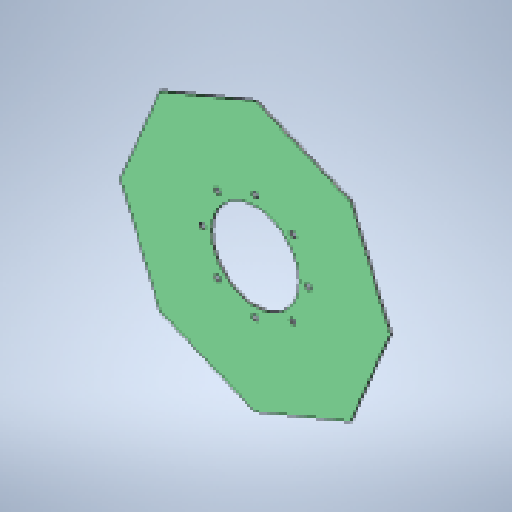
# Autodesk Inventor part: DMF 01 21 Барабан торец НОС v2.1_наруж
Saved by Autodesk Inventor 2026.2 (Build 302298010, 298A)
## iProperties
Created: 2024-04-28
Part Number: DMF 01 21 Барабан торец НОС v2.1_наруж
Material: Generic
Document SubType Name: Sheet Metal
Designer: admin
Stock Number: Барабан_Торец_Нос
Density: 1 g/cm^3
Flat Pattern Width: 51.5 cm
Flat Pattern Length: 51.5 cm
Flat Pattern Area: 2652.25 cm^2
Sheet Metal Rule: Default
Sheet Metal Width: 515,000 mm
Sheet Metal Length: 515,000 mm
Sheet Metal Area: 265225,000 mm^2
Appearance: Default
Author: pokla
Autodesk Inventor part; units mm, degrees
ref_plane "YZ Plane" through (0, 0, 0) normal (1, 0, 0) x (0, 1, 0)
ref_plane "XZ Plane" through (0, 0, 0) normal (0, 1, 0) x (-1, 0, 0)
ref_plane "XY Plane" through (0, 0, 0) normal (0, 0, 1) x (1, 0, 0)
sketch "Sketch2" plane through (0, 0, 0) normal (0, 0, 1) x (1, 0, 0)
  line L0 (-197.082, 197.082) -> (0, 278.716)
  line L1 (0, 278.716) -> (197.082, 197.082)
  line L2 (197.082, 197.082) -> (278.716, 0)
  line L3 (278.716, 0) -> (197.082, -197.082)
  line L4 (197.082, -197.082) -> (0, -278.716)
  line L5 (0, -278.716) -> (-197.082, -197.082)
  line L6 (-197.082, -197.082) -> (-278.716, 0)
  line L7 (-278.716, 0) -> (-197.082, 197.082)
  circle A0 centre (0, 0) radius 90
  dimension "d23" = 515
  dimension "d26" = 180
  measures "d23" distance between parallel lines of L6 L2
  measures "d26" diameter of A0
extrude "Plate1" add sketch "Sketch2" against normal blind 3
sketch "Sketch4" plane through (0, 0, 0) normal (0, 0, 1) x (1, 0, 0)
  circle A0 centre (0, 110) radius 6.25
  circle A1 centre (0, 0) radius 90 projected
  circle A2 centre (0, 0) radius 110 construction
  dimension "d28" = 220
  dimension "d16" = 12.5
  constraints: 2 vertical alignment, 1 centre point, 1 coincident, 2 other
  measures "d16" diameter of A0
extrude "Extrusion1" cut sketch "Sketch4" against normal up to surface (3 mm away) contours A0
pattern_circular "Circular Pattern1" count 8 over 360 about axis through (0, 0, -10) along (0, 0, 1) of "Extrusion1"
equation "\"d23\" = Барабан_размер_по_плоскостям"
equation "\"d15\" = Thickness"
equation "\"BendRadius\" = Thickness"
equation "\"BendReliefWidth\" = Thickness"
equation "\"BendReliefDepth\" = 0.5 * Thickness"
equation "\"CornerReliefSize\" = 4 * Thickness"
equation "\"MinimumRemnant\" = 2 * Thickness"
equation "\"TransitionRadius\" = BendRadius"
equation "\"JacobiRadiusSize\" = BendRadius"
equation "\"GapSize\" = Thickness"
equation "\"Барабан_размер_по_плоскостям\" = 515"
equation "\"Thickness\" = 3"
body "Solid1"
